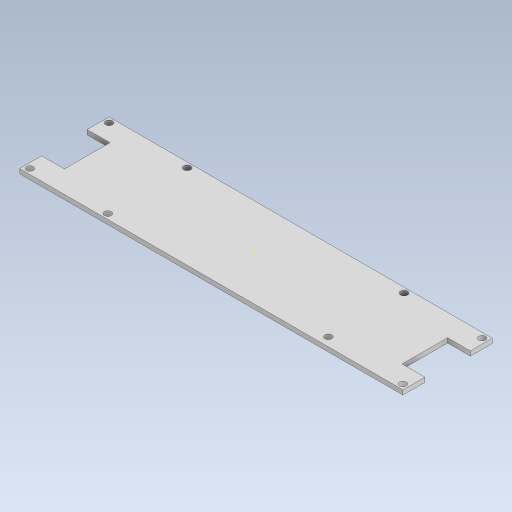
# Autodesk Inventor part: Casis Tengah
Saved by Autodesk Inventor 2023.5 (Build 275446000, 446)
## iProperties
Created: 2025-09-06
Part Number: Casis Tengah
Material: Generic
Document SubType Name: Modeling
Designer: Guntur
Density: 1 g/cm^3
Appearance: Default
Author: Guntur
## iProperties of the stored document Casis Tengah_3DPrint.ipt
Created: 2025-09-06
Part Number: Casis Tengah_3DPrint
Material: Generic
Document SubType Name: Modeling
Designer: Guntur
Density: 1 g/cm^3
Appearance: Default
Author: Guntur
Autodesk Inventor part; units mm, degrees
ref_plane "YZ Plane" through (0, 0, 0) normal (1, 0, 0) x (0, 1, 0)
ref_plane "XZ Plane" through (0, 0, 0) normal (0, 1, 0) x (-1, 0, 0)
ref_plane "XY Plane" through (0, 0, 0) normal (0, 0, 1) x (1, 0, 0)
sketch "Sketch1" plane through (0, 0, 0) normal (0, 1, 0) x (-1, 0, 0)
  line L0 (83.5, 19.65) -> (-85, 19.65)
  line L1 (-85, 19.65) -> (-85, -19.65)
  line L2 (-85, -19.65) -> (83.5, -19.65)
  line L3 (83.5, -19.65) -> (83.5, 19.65)
  line L4 (19.05, 0) -> (-17.4625, 0) construction
  line L5 (-0.75, 11.1125) -> (-0.75, -12.7) construction
  circle A0 centre (-82.75, 17.4) radius 1.5
  circle A1 centre (-82.75, -17.4) radius 1.5
  circle A2 centre (81.25, 17.4) radius 1.5
  circle A3 centre (81.25, -17.4) radius 1.5
  circle A4 centre (46.95, 17.4) radius 1.5
  circle A5 centre (46.95, -17.4) radius 1.5
  circle A6 centre (-48.45, -17.4) radius 1.5
  circle A7 centre (-48.45, 15.9) radius 1.5
  point P0 (0, 0)
  dimension "d0" = 168.5
  dimension "d1" = 39.3
  dimension "d2" = 3
  dimension "d3" = 2.25
  dimension "d4" = 2.25
  dimension "d7" = 2.25
  dimension "d16" = 3
  dimension "d17" = 34.3
  dimension "d18" = 3
  dimension "d19" = 3
  dimension "d20" = 34.3
  dimension "d21" = 3
  constraints: 12 end point, 8 centre point, 3 symmetric about line, 2 horizontal, 2 parallel, 1 perpendicular, 1 vertical, 3 other
  measures "d0" distance of L2.end L1.end
  measures "d1" distance of L1.end L0.end
  measures "d2" diameter of A0
  measures "d3" distance from line of L0 A0.centre
  measures "d4" distance from line of L1 A0.centre
  measures "d7" distance from line of L3 A2.centre
  measures "d16" diameter of A4
  measures "d17" distance of A2.centre A4.centre
  measures "d18" diameter of A5
  measures "d19" diameter of A6
  measures "d20" distance of A1.centre A6.centre
  measures "d21" diameter of A7
extrude "Extrusion1" add sketch "Sketch1" along normal blind 2 contours L3 L2 L1 L0 | A2 | A3 | A4 | A5 | A6 | A7
extrude "Extrusion2" cut sketch "Sketch1" along normal blind 2 contours A2 | A3
sketch "Sketch2" plane through (0, 2, 0) normal (0, 1, 0) x (1, 0, 0)
  line L0 (-93.5, -10) -> (-73.5, -10)
  line L1 (-73.5, -10) -> (-73.5, 10)
  line L2 (-73.5, 10) -> (-93.5, 10)
  line L3 (-93.5, 10) -> (-93.5, -10)
  line L4 (-83.5, 19.65) -> (-83.5, -19.65) projected
  line L5 (-93.5, -10) -> (-73.5, 10) construction
  line L6 (-73.5, -10) -> (-93.5, 10) construction
  line L7 (75, -10) -> (95, -10)
  line L8 (95, -10) -> (95, 10)
  line L9 (95, 10) -> (75, 10)
  line L10 (75, 10) -> (75, -10)
  line L11 (85, -19.65) -> (85, 19.65) projected
  line L12 (75, -10) -> (95, 10) construction
  line L13 (95, -10) -> (75, 10) construction
  point P0 (0, 0)
  point P1 (-83.5, 0)
  point P2 (85, 0)
  point P3 (-83.5, 10)
  point P4 (-83.5, -10)
  point P5 (85, -10)
  point P6 (85, 10)
  dimension "d10" = 20
  dimension "d11" = 20
  dimension "d12" = 20
  dimension "d13" = 20
  constraints: 24 end point, 6 midpoint, 4 parallel, 2 horizontal, 2 perpendicular
  measures "d10" distance of L2.end L1.end
  measures "d11" distance of L1.end L0.end
  measures "d12" distance of L9.end L8.end
  measures "d13" distance of L8.end L7.end
extrude "Extrusion3" cut sketch "Sketch2" against normal blind 2 contours L4 L2 L1 L0 | L10 L9 L11 L7
sketch "Sketch3" plane through (0, 2, 0) normal (0, 1, 0) x (1, 0, 0)
  point P0 (0, 0)
extrude "Extrusion4" cut sketch "Sketch1" along normal blind 2 contours A4 | A5 | A6 | A7
body "Solid1"
